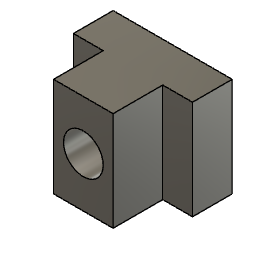
bed-screw-plate (Autodesk Fusion 360 design; units mm, degrees)
Autodesk Fusion 360 part; units mm, degrees
sketch "Sketch1" plane through (0, 0, 0) normal (0, 0, 1) x (1, 0, 0)
  line L0 (-6, 5) -> (6, 5)
  line L1 (6, 5) -> (6, -5)
  line L2 (6, -5) -> (-6, -5)
  line L3 (-6, -5) -> (-6, 5)
  line L4 (-3, 5) -> (3, 5)
  line L5 (3, 5) -> (3, -5)
  line L6 (3, -5) -> (-3, -5)
  line L7 (-3, -5) -> (-3, 5)
  circle A0 centre (0, 0) radius 2
  dimension "d1" = 4
  dimension "d2" = 12
  dimension "d3" = 10
  dimension "d4" = 6
  constraint horizontal L0
  constraint vertical L1
  constraint horizontal L2
  constraint vertical L3
  constraint horizontal L4
  constraint vertical L5
  constraint horizontal L6
  constraint vertical L7
  constraint coincident L2 L5.end
  constraint coincident A0.centre origin
  measures "d1" diameter of A0
  measures "d2" distance of L0.start L0.end
  measures "d3" distance of L0.start L2.end
  measures "d4" distance of L5.end L6.end
extrude "Extrude1" add sketch "Sketch1" along normal blind 9 contours L0 L2 L4 L5 L6 L7
extrude "Extrude2" add sketch "Sketch1" along normal blind 4 contours L0 L2 L3 L7 | L0 L1 L2 L5
